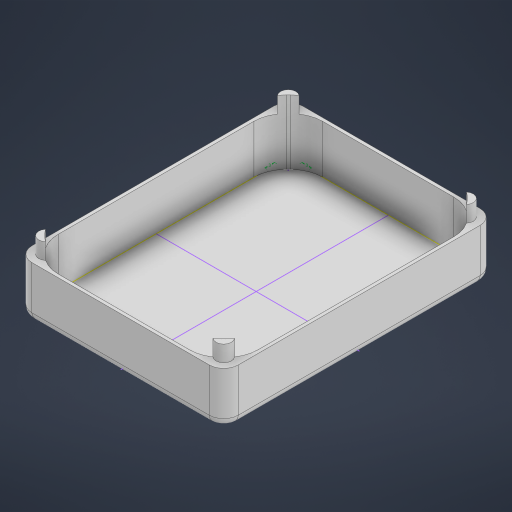
# Autodesk Inventor part: ShadeV2
Saved by Autodesk Inventor 2024 (Build 280153000, 153)
## iProperties
Created: 2023-08-04
Part Number: ShadeV2
Material: Generic
Document SubType Name: Modeling
Designer: Noah
Density: 1 g/cm^3
Appearance: Default
Author: Noah
## iProperties of the stored document ShadeV2_3DPrint.ipt
Created: 2023-08-05
Part Number: ShadeV2_3DPrint
Material: Generic
Document SubType Name: Modeling
Designer: Noah
Density: 1 g/cm^3
Appearance: Default
Author: Noah
Autodesk Inventor part; units mm, degrees
ref_plane "YZ Plane" through (0, 0, 0) normal (1, 0, 0) x (0, 1, 0)
ref_plane "XZ Plane" through (0, 0, 0) normal (0, 1, 0) x (-1, 0, 0)
ref_plane "XY Plane" through (0, 0, 0) normal (0, 0, 1) x (1, 0, 0)
sketch "Sketch1" plane through (0, 0, 0) normal (0, 1, 0) x (-1, 0, 0)
  line L0 (0, -48.25) -> (0, -79.5)
  arc A0 (0, -79.5) -> (4.5, -84) centre (4.5, -79.5) ccw
  line L1 (4.5, -84) -> (59.5, -84)
  arc A1 (59.5, -84) -> (64, -79.5) centre (59.5, -79.5) ccw
  line L2 (64, -79.5) -> (64, -4.5)
  arc A2 (64, -4.5) -> (59.5, 0) centre (59.5, -4.5) ccw
  line L3 (59.5, 0) -> (4.5, 0)
  arc A3 (4.5, 0) -> (0, -4.5) centre (4.5, -4.5) ccw
  line L4 (0, -4.5) -> (0, -35.75)
  line L5 (2, -35.75) -> (2, -4.5)
  arc A4 (4.5, -2) -> (2, -4.5) centre (4.5, -4.5) ccw
  line L6 (4.5, -2) -> (59.5, -2)
  arc A5 (62, -4.5) -> (59.5, -2) centre (59.5, -4.5) ccw
  line L7 (62, -4.5) -> (62, -79.5)
  arc A6 (59.5, -82) -> (62, -79.5) centre (59.5, -79.5) ccw
  line L8 (59.5, -82) -> (4.5, -82)
  arc A7 (2, -79.5) -> (4.5, -82) centre (4.5, -79.5) ccw
  line L9 (2, -79.5) -> (2, -48.25)
  line L10 (2, -35.75) -> (2, -48.25)
  line L11 (0, -48.25) -> (0, -35.75)
  line L12 (4.5, -1) -> (59.5, -1)
  arc A8 (63, -4.5) -> (59.5, -1) centre (59.5, -4.5) ccw
  line L13 (63, -4.5) -> (63, -79.5)
  arc A9 (59.5, -83) -> (63, -79.5) centre (59.5, -79.5) ccw
  line L14 (59.5, -83) -> (4.5, -83)
  arc A10 (1, -79.5) -> (4.5, -83) centre (4.5, -79.5) ccw
  line L15 (1, -79.5) -> (1, -48.25)
  line L16 (1, -48.25) -> (1, -35.75)
  line L17 (1, -35.75) -> (1, -4.5)
  arc A11 (4.5, -1) -> (1, -4.5) centre (4.5, -4.5) ccw
  point P0 (0, 0)
  point P1 (57, -77)
  point P2 (0, 0)
  dimension "d0" = 1
  constraints: 36 end point, 24 point on circle, 12 centre point, 3 collinear, 9 other
  measures "d0" distance between parallel lines of L3 L12
extrude "Extrusion1" add sketch "Sketch1" along normal blind 15 contours L11 L4 A3 L3 A2 L2 A1 L1 A0 L0
sketch "Sketch2" plane through (0, 0, 0) normal (0, -1, 0) x (1, 0, 0)
  arc A0 (-4.5, -84) -> (0, -79.5) centre (-4.5, -79.5) ccw projected
  line L0 (0, -4.5) -> (0, -79.5) projected
  arc A1 (0, -4.5) -> (-4.5, 0) centre (-4.5, -4.5) ccw projected
  line L1 (-59.5, 0) -> (-4.5, 0) projected
  arc A2 (-59.5, 0) -> (-64, -4.5) centre (-59.5, -4.5) ccw projected
  line L2 (-64, -79.5) -> (-64, -4.5) projected
  arc A3 (-64, -79.5) -> (-59.5, -84) centre (-59.5, -79.5) ccw projected
  line L3 (-4.5, -84) -> (-59.5, -84) projected
  line L4 (-1, -79.5) -> (-1, -4.5) projected
  arc A4 (-4.5, -83) -> (-1, -79.5) centre (-4.5, -79.5) ccw projected
  line L5 (-59.5, -83) -> (-4.5, -83) projected
  arc A5 (-63, -79.5) -> (-59.5, -83) centre (-59.5, -79.5) ccw projected
  line L6 (-63, -4.5) -> (-63, -79.5) projected
  arc A6 (-59.5, -1) -> (-63, -4.5) centre (-59.5, -4.5) ccw projected
  line L7 (-4.5, -1) -> (-59.5, -1) projected
  arc A7 (-1, -4.5) -> (-4.5, -1) centre (-4.5, -4.5) ccw projected
  point P0 (0, 0)
extrude "Extrusion2" add sketch "Sketch2" along normal blind 1 contours L3 A3 L2 A2 L1 A1 L0 A0 | A4 L5 A5 L6 A6 L7 A7 L4
fillet "Fillet1" radius 2.5 8 edges at (-64, -1, -42) (-62.682, -1, -82.682) (-32, -1, -84) (-1.318, -1, -82.682) (0, -1, -42) (-1.318, -1, -1.318) (-32, -1, 0) (-62.682, -1, -1.318)
sketch "Sketch3" plane through (0, 0, 0) normal (0, 1, 0) x (1, 0, 0)
  line L0 (-63, 4.5) -> (-63, 79.5) projected
  line L1 (-63, 42) -> (0, 42)
  line L2 (-59.5, 84) -> (-4.5, 84) projected
  line L3 (-32, 84) -> (-32, 0)
  arc A0 (-59.5, 81.875) -> (-61.875, 79.5) centre (-59.5, 79.5) ccw
  arc A1 (-1, 79.5) -> (-4.5, 83) centre (-4.5, 79.5) ccw projected
  line L4 (-59.5, 83) -> (-4.5, 83) projected
  arc A2 (-59.5, 83) -> (-63, 79.5) centre (-59.5, 79.5) ccw projected
  line L5 (-63, 4.5) -> (-63, 79.5) projected
  arc A3 (-63, 4.5) -> (-59.5, 1) centre (-59.5, 4.5) ccw projected
  line L6 (-4.5, 1) -> (-59.5, 1) projected
  arc A4 (-4.5, 1) -> (-1, 4.5) centre (-4.5, 4.5) ccw projected
  line L7 (-1, 79.5) -> (-1, 4.5) projected
  arc A5 (-58.0893, 81.4107) -> (-61.4107, 78.0893) centre (-59.5, 79.5) ccw
  line L8 (-63, 79.5) -> (-63, 76.5)
  line L9 (-59.5, 83) -> (-56.5, 83)
  line L10 (-59.5, 83) -> (-4.5, 83) projected
  line L11 (-56.5, 83) -> (-63, 76.5)
  arc A6 (-2.5893, 78.0893) -> (-5.9107, 81.4107) centre (-4.5, 79.5) ccw
  line L12 (-7.5, 83) -> (-1, 76.5)
  arc A7 (-61.4107, 5.9107) -> (-58.0893, 2.5893) centre (-59.5, 4.5) ccw
  line L13 (-56.5, 1) -> (-63, 7.5)
  line L14 (-7.5, 1) -> (-1, 7.5)
  arc A8 (-5.9107, 2.5893) -> (-2.5893, 5.9107) centre (-4.5, 4.5) ccw
  point P0 (-59.5, 4.5)
  point P1 (-1, 42)
  point P2 (-1, 7.5)
  dimension "d17" = 3
  dimension "d18" = 3
  constraints: 17 symmetric about line, 16 end point, 10 point on circle, 10 point on line, 5 centre point, 2 midpoint, 1 coincident, 1 concentric, 3 other
  measures "d17" distance of L5.end L8.end
  measures "d18" distance of L4.start L9.end
extrude "Extrusion5" add sketch "Sketch3" along normal up to surface (15 mm away) contours L0 L13 A7 L6 A3 | L0 A2 L4 L11 A5 A0 | L14 A8 L7 A4 L6 | L12 A6 L4 A1 L7
extrude "Extrusion6" add sketch "Sketch3" along normal blind 20 contours L13 A7 | A5 A0 L11 | L14 A8 | L12 A6
fillet "Fillet3" radius 10 8 edges at (-63, 7.5, -7.5) (-56.5, 7.5, -1) (-63, 7.5, -76.5) (-56.5, 7.5, -83) (-7.5, 7.5, -83) (-1, 7.5, -76.5) (-1, 7.5, -7.5) (-7.5, 7.5, -1)
body "Solid1"
